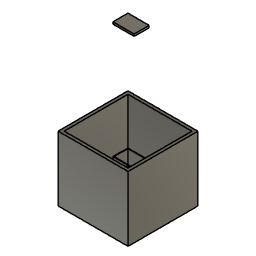
greenlight v2 (Autodesk Fusion 360 design; units mm, degrees)
Autodesk Fusion 360 part; units mm, degrees
note: some values were not read from the file. Chosen so that the rebuilt part matches the saved one: which bodies a step acts on; which face or edge a step refers to.
sketch "Sketch1" plane through (0, 0, 0) normal (0, 0, 1) x (1, 0, 0)
  line L0 (-48.4645, 25.1958) -> (91.7437, 25.1958)
  line L1 (91.7437, 25.1958) -> (91.7437, -114.8042)
  line L2 (91.7437, -114.8042) -> (-48.4645, -114.8042)
  line L3 (-48.4645, -114.8042) -> (-48.4645, 25.1958)
  dimension "d1" = 140
  constraint horizontal L0
  constraint vertical L1
  constraint horizontal L2
  constraint vertical L3
  measures "d1" distance of L0.start L2.end
extrude "Extrude1" add sketch "Sketch1" along normal blind 140 makes body 1
sketch "Sketch2" plane through (0, 0, 0) normal (1, 0, 0) x (0, 1, 0)
  line L0 (30, 130) -> (-165.3892, 130)
  constraint horizontal L0
split "Split1" by curves path "Sketch2" along L0 bodies 1 makes body 2 at (45.0076, -68.1375, 140)
move_body "Move1" bodies 2 to x (1, 0, 0) y (0, 1, 0) z (0, 0, 1) at (0, 0, 100)
shell "Shell1" thickness 6 removed faces 1 at (45.0076, -21.4708, 130) on bodies 1
sketch "Sketch3" plane through (0, 0, 240) normal (0, 0, 1) x (-1, 0, 0)
  line L0 (-80.4193, 68.8311, -220) -> (-63.8424, 68.8311, -220)
  line L1 (-63.8424, 68.8311, -220) -> (-63.8424, 32.8311, -220)
  line L2 (-63.8424, 32.8311, -220) -> (-80.4193, 32.8311, -220)
  line L3 (-80.4193, 32.8311, -220) -> (-80.4193, 68.8311, -220)
  line L4 (7.5895, 106.4876, -220) -> (7.5895, 89.9107, -220)
  line L5 (-28.4105, 106.4876, -220) -> (7.5895, 106.4876, -220)
  line L6 (-28.4105, 89.9107, -220) -> (-28.4105, 106.4876, -220)
  line L7 (7.5895, 89.9107, -220) -> (-28.4105, 89.9107, -220)
  dimension "d5" = 36
  dimension "d6" = 36
sketch "Sketch4" plane through (0, 0, 6) normal (0, 0, 1) x (-1, 0, 0)
  line L0 (42.4645, 108.8042) -> (-85.7437, 108.8042)
  line L1 (-85.7437, 108.8042) -> (-85.7437, -19.1958)
  line L2 (-85.7437, -19.1958) -> (42.4645, -19.1958)
  line L3 (42.4645, -19.1958) -> (42.4645, 108.8042)
  line L4 (-25.7071, 65) -> (-21.3336, 65)
  line L5 (-21.3336, 65) -> (-21.3336, 34.8025)
  line L6 (-21.3336, 34.8025) -> (-25.7071, 34.8025)
  line L7 (-25.7071, 34.8025) -> (-25.7071, 65)
  constraint horizontal L4
  constraint vertical L5
  constraint horizontal L6
  constraint vertical L7
extrude "Extrude2" add sketch "Sketch4" along normal blind 55 separate body contours L4 L5 L6 L7 makes body 3
move_body "Move2" bodies 3 to x (0.707107, 0.707107, 0) y (-0.707107, 0.707107, 0) z (0, 0, 1) at (-29.0371, -29.7009, 0)
sketch "Sketch5" plane through (-11.1913, -11.1913, 0) normal (0.707107, 0.707107, 0) x (-0.707107, 0.707107, 0)
  line L0 (-65.4694, 6) -> (-35.2719, 6)
  line L1 (-35.2719, 6) -> (-35.2719, 61)
  line L2 (-35.2719, 61) -> (-65.4694, 61)
  line L3 (-65.4694, 61) -> (-65.4694, 6)
  line L4 (-63.0538, 54.3494) -> (-37.7036, 54.3494)
  line L5 (-37.7036, 54.3494) -> (-37.7036, 11.4177)
  line L6 (-37.7036, 11.4177) -> (-63.0538, 11.4177)
  line L7 (-63.0538, 11.4177) -> (-63.0538, 54.3494)
  constraint horizontal L4
  constraint vertical L5
  constraint horizontal L6
  constraint vertical L7
extrude "Extrude3" cut sketch "Sketch5" against normal blind 25 contours L4 L5 L6 L7 bodies 3
sketch "Sketch3 (curves -220 mm off its plane)" plane through (0, 0, 20) normal (0, 0, 1) x (-1, 0, 0)
  line L0 (-80.4193, 68.8311) -> (-63.8424, 68.8311)
  line L1 (-63.8424, 68.8311) -> (-63.8424, 32.8311)
  line L2 (-63.8424, 32.8311) -> (-80.4193, 32.8311)
  line L3 (-80.4193, 32.8311) -> (-80.4193, 68.8311)
  line L4 (7.5895, 106.4876) -> (7.5895, 89.9107)
  line L5 (-28.4105, 106.4876) -> (7.5895, 106.4876)
  line L6 (-28.4105, 89.9107) -> (-28.4105, 106.4876)
  line L7 (7.5895, 89.9107) -> (-28.4105, 89.9107)
extrude "Extrude4" cut sketch "Sketch3 (curves -220 mm off its plane)" against normal blind 16 bodies 1
sketch "Sketch6" plane through (0, 0, 6) normal (0, 0, 1) x (-1, 0, 0)
  line L0 (-28.4105, 106.4876) -> (7.5895, 106.4876)
  line L1 (7.5895, 106.4876) -> (7.5895, 89.9107)
  line L2 (7.5895, 89.9107) -> (-28.4105, 89.9107)
  line L3 (-28.4105, 89.9107) -> (-28.4105, 106.4876)
  line L4 (-63.8424, 68.8311) -> (-63.8424, 32.8311)
  line L5 (-63.8424, 32.8311) -> (-80.4193, 32.8311)
  line L6 (-80.4193, 32.8311) -> (-80.4193, 68.8311)
  line L7 (-80.4193, 68.8311) -> (-63.8424, 68.8311)
  line L8 (42.4645, 108.8042) -> (-85.7437, 108.8042)
  line L9 (-85.7437, 108.8042) -> (-85.7437, -19.1958)
  line L10 (-85.7437, -19.1958) -> (42.4645, -19.1958)
  line L11 (42.4645, -19.1958) -> (42.4645, 108.8042)
  line L12 (10, 70) -> (14, 70)
  line L13 (14, 70) -> (14, 40)
  line L14 (14, 40) -> (10, 40)
  line L15 (10, 40) -> (10, 70)
  constraint horizontal L12
  constraint vertical L13
  constraint horizontal L14
  constraint vertical L15
extrude "Extrude5" add sketch "Sketch6" along normal blind 36 separate body contours L12 L13 L14 L15 makes body 4
hole "Hole1" at (-10, -55, 24) direction (-1, 0, 0) diameter 27 depth 13 tip angle 118 bodies 4
sketch "Sketch7" plane through (0, 0, 6) normal (0, 0, 1) x (-1, 0, 0)
  line L0 (-28.4105, 106.4876) -> (7.5895, 106.4876)
  line L1 (7.5895, 106.4876) -> (7.5895, 89.9107)
  line L2 (7.5895, 89.9107) -> (-28.4105, 89.9107)
  line L3 (-28.4105, 89.9107) -> (-28.4105, 106.4876)
  line L4 (-63.8424, 68.8311) -> (-63.8424, 32.8311)
  line L5 (-63.8424, 32.8311) -> (-80.4193, 32.8311)
  line L6 (-80.4193, 32.8311) -> (-80.4193, 68.8311)
  line L7 (-80.4193, 68.8311) -> (-63.8424, 68.8311)
  line L8 (42.4645, 108.8042) -> (-85.7437, 108.8042)
  line L9 (-85.7437, 108.8042) -> (-85.7437, -19.1958)
  line L10 (-85.7437, -19.1958) -> (42.4645, -19.1958)
  line L11 (42.4645, -19.1958) -> (42.4645, 108.8042)
  line L12 (32, 70) -> (38, 70)
  line L13 (38, 70) -> (38, 40)
  line L14 (38, 40) -> (32, 40)
  line L15 (32, 40) -> (32, 70)
  constraint horizontal L12
  constraint vertical L13
  constraint horizontal L14
  constraint vertical L15
extrude "Extrude6" add sketch "Sketch7" along normal blind 38 separate body contours L12 L13 L14 L15 makes body 5
hole "Hole2" at (-32, -54.1381, 33.587) direction (-1, 0, 0) diameter 15 depth 6 tip angle 118 bodies 1 5
sketch "Sketch8" plane through (0, 0, 6) normal (0, 0, 1) x (-1, 0, 0)
  line L0 (-28.4105, 106.4876) -> (7.5895, 106.4876)
  line L1 (7.5895, 106.4876) -> (7.5895, 89.9107)
  line L2 (7.5895, 89.9107) -> (-28.4105, 89.9107)
  line L3 (-28.4105, 89.9107) -> (-28.4105, 106.4876)
  line L4 (-63.8424, 68.8311) -> (-63.8424, 32.8311)
  line L5 (-63.8424, 32.8311) -> (-80.4193, 32.8311)
  line L6 (-80.4193, 32.8311) -> (-80.4193, 68.8311)
  line L7 (-80.4193, 68.8311) -> (-63.8424, 68.8311)
  line L8 (42.4645, 108.8042) -> (-85.7437, 108.8042)
  line L9 (-85.7437, 108.8042) -> (-85.7437, -19.1958)
  line L10 (-85.7437, -19.1958) -> (42.4645, -19.1958)
  line L11 (42.4645, -19.1958) -> (42.4645, 108.8042)
  line L12 (42.4645, -19.1958) -> (0, -19.1958)
  line L13 (0, -19.1958) -> (0, 11)
  line L14 (0, 11) -> (42.4645, 11)
  line L15 (42.4645, 11) -> (42.4645, -19.1958)
  constraint horizontal L12
  constraint vertical L13
  constraint horizontal L14
  constraint vertical L15
  constraint coincident L10.end L11.start
extrude "Extrude7" add sketch "Sketch8" along normal blind 35 separate body contours L10 L11 L12 L13 L14 L15 makes body 6
sketch "Sketch9" plane through (0, 0, 0) normal (1, 0, 0) x (0, 1, 0)
  line L0 (-11, 6) -> (19.1958, 6)
  line L1 (19.1958, 6) -> (19.1958, 41)
  line L2 (19.1958, 41) -> (-11, 41)
  line L3 (-11, 41) -> (-11, 6)
  line L4 (-11, 37) -> (19.1958, 36.5421)
  constraint coincident L3 L4.start
  constraint coincident L1 L4.end
split "Split2" by curves path "Sketch9" along L4 bodies 6 makes body 7 at (-14.1548, -11, 16.3333)
move_body "Move3" bodies 6 to x (1, 0, 0) y (0, 1, 0) z (0, 0, 1) at (0, 0, 130)
shell "Shell2" thickness 1 removed faces 1 at (-28.3097, -0.9347, 36.8474) on bodies 7
hole "Hole3" at (-41.4645, 3.5856, 10.6332) direction (-1, 0, 0) diameter 7 depth 15 tip angle 118 bodies 1 7
hole "Hole4" at (-38.4498, -11, 9.3454) direction (0, 1, 0) diameter 4 depth 15 tip angle 118 bodies 7
hole "Hole5" at (0, 5.6497, 11.0831) direction (-1, 0, 0) diameter 7 depth 15 tip angle 118 bodies 7
move_body "Move4" bodies 2 to x (1, 0, 0) y (0, 1, 0) z (0, 0, 1) at (0, 0, 140)
move_body "Move5" bodies 6 to x (1, 0, 0) y (0, 1, 0) z (0, 0, 1) at (0, 0, 100)
other "Base Mesh Feature1"
other "CopyPasteMeshes1"
other "Modify1"
other "Modify2"
other "Modify3"
hidden bodies 2
